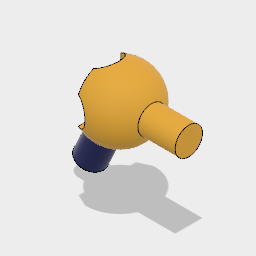
Ball_joint (Autodesk Fusion 360 design; units mm, degrees)
Autodesk Fusion 360 part; units mm, degrees
note: some values were not read from the file. Chosen so that the rebuilt part matches the saved one: which face or edge a step refers to.
cylinder "CylinderPrimitive1" add diameter 20 height 50 placed x (1, 0, 0) y (0, 0, -1) z (0, 1, 0) at (0, 0, 0) makes body 1
sphere "SpherePrimitive1" add diameter 40 placed x (-1, 0, 0) y (0, 0, 1) z (0, 1, 0) at (0, 50, 0) bodies 1
ref_plane "WorkPlane1" through (0, 33, 0) normal (0, -1, 0) x (-1, 0, 0)
copy_body "CopyPasteBodies2" bodies 1 makes body 2
move_body "Move2" bodies 2 to x (0, -1, 0) y (1, 0, 0) z (0, 0, 1) at (-50, 50, 0)
copy_body "Body->Comp1" bodies 2 removing the originals makes body 3 in component "Component"
copy_body "Body->Comp2" bodies 1 removing the originals makes body 4 in component "Component'"
move_body "Move1" bodies 4 to x (1, 0, 0) y (0, 1, 0) z (0, 0, 1) at (20, 0, 0) in component "Component'"
move_body "Move2'" bodies 4 to x (0, 1, 0) y (-1, 0, 0) z (0, 0, 1) at (70, 30, 0) in component "Component'"
move_face "OffsetFaces1" offset 5 1 faces at (14.8236, 30.975, 3.3546) on bodies 4 in component "Component'"
combine "Combine1" operation cut target body 4 tool bodies 3 body 3 seen with x (1, 0, 0) y (0, 1, 0) z (0, 0, 1) at (20, 0, 0) keep tools in component "Component'"
ref_plane "WorkPlane2" through (0.2472, 42.3428, 6.4317) normal (0, 0.765721, -0.643173) x (0, -0.643173, -0.765721)
sketch "Sketch12" plane through (0.2472, 42.3428, 6.4317) normal (0, 0.765721, -0.643173) x (0, -0.643173, -0.765721)
  line L0 (-35, -10.2598) -> (35, -10.2598)
  line L1 (35, -10.2598) -> (35, 15)
  line L2 (35, 15) -> (-35, 15)
  line L3 (-35, 15) -> (-35, -10.2598)
extrude "Extrude1" cut sketch "Sketch12" along normal mid plane 70 bodies 4 in component "Component'"
move_face "OffsetFaces1'" offset -0.8 1 faces at (5.1764, 69.025, 3.3546) on bodies 3 in component "Component"
combine "Combine3" operation cut target body 4 tool bodies 3 body 3 seen with x (0.422618, 0.906308, 0) y (-0.906308, 0.422618, 0) z (0, 0, 1) at (65.3154, 28.8691, 0) keep tools in component "Component'"
pattern_circular "C-Pattern2" count 4 over 360 about axis through (42.9129, 50, 0) along (1, 0, 0) of 1 faces at (11.8849, 31.0781, 9.9794) on bodies 4 in component "Component'"
component "Component" placed x (0.422618, 0.906308, 0) y (-0.906308, 0.422618, 0) z (0, 0, 1) at (65.3154, 28.8691, 0)
component "Component'" placed x (1, 0, 0) y (0, 1, 0) z (0, 0, 1) at (0, 0, 0)
